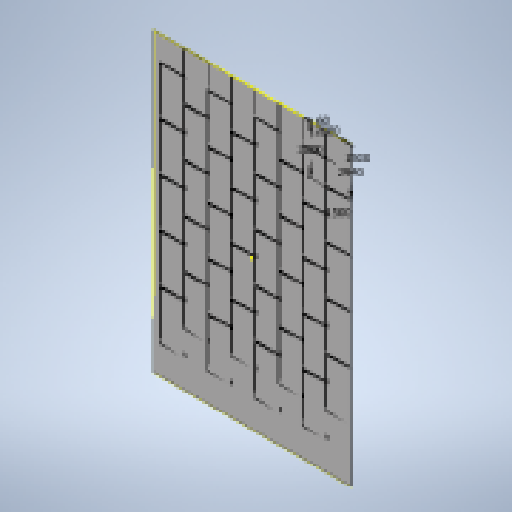
# Autodesk Inventor part: Part1
Saved by Autodesk Inventor 2026.2 (Build 302298000, 298)
## iProperties
Created: 2026-04-17
Part Number: Part1
Material: Generic
Document SubType Name: Sheet Metal
Designer: admin
Density: 1 g/cm^3
Sheet Metal Rule: Default_mm
Appearance: Default
Author: admin
Autodesk Inventor part; units mm, degrees
ref_plane "YZ Plane" through (0, 0, 0) normal (1, 0, 0) x (0, 1, 0)
ref_plane "XZ Plane" through (0, 0, 0) normal (0, 1, 0) x (-1, 0, 0)
ref_plane "XY Plane" through (0, 0, 0) normal (0, 0, 1) x (1, 0, 0)
sketch "Sketch1" plane through (0, 0, 0) normal (0, 0, 1) x (1, 0, 0)
  line L0 (6000, -9000) -> (-6000, -9000)
  line L1 (-6000, -9000) -> (-6000, 9000)
  line L2 (-6000, 9000) -> (6000, 9000)
  line L3 (6000, 9000) -> (6000, -9000)
  line L4 (6000, -9000) -> (-6000, 9000) construction
  line L5 (-6000, -9000) -> (6000, 9000) construction
  point P0 (0, 0)
  dimension "d0" = 12000
  dimension "d1" = 18000
  measures "d0" distance of L1.end L2.end
  measures "d1" distance of L0.end L1.end
extrude "Plate1" add sketch "Sketch1" along normal blind 6
sketch "Sketch2" plane through (0, 0, 6) normal (0, 0, 1) x (1, 0, 0)
  line L0 (6000, 9000) -> (6000, -9000)
  line L1 (-6000, 9000) -> (6000, 9000) projected
  line L2 (-6000, -9000) -> (-6000, 9000) projected
  line L3 (6000, -9000) -> (-6000, -9000) projected
  line L4 (5800, -8800) -> (5800, 8800)
  line L5 (5800, 8800) -> (-5800, 8800)
  line L6 (-5800, 8800) -> (-5800, -8800)
  line L7 (-5800, -8800) -> (5800, -8800)
  line L8 (6000, 9000) -> (-6000, 9000) projected
  line L9 (6000, 9000) -> (4500, 9000)
  line L10 (4500, 9000) -> (4500, 6000)
  line L11 (4500, 6000) -> (6000, 6000)
  line L12 (6000, 6000) -> (6000, 9000)
  line L13 (6000, -9000) -> (6000, 9000) projected
  line L14 (6000, 5975.1164) -> (4500, 5975.1164)
  line L15 (4500, 5975.1164) -> (4500, 2838.9347)
  line L16 (4500, 2838.9347) -> (6000, 2838.9347)
  line L17 (6000, 2838.9347) -> (6000, 5975.1164)
  line L18 (4448.9335, 7446.1559) -> (3367.2381, 7446.1559)
  line L19 (3367.2381, 7446.1559) -> (3367.2381, 4345.2957)
  line L20 (3367.2381, 4345.2957) -> (4448.9335, 4345.2957)
  line L21 (4448.9335, 4345.2957) -> (4448.9335, 7446.1559)
  line L22 (6000, 6064.0733) -> (4383.2518, 6064.0733) construction
  line L23 (4383.2518, 6064.0733) -> (4383.2518, 5895.7258) construction
  line L24 (4383.2518, 5895.7258) -> (6000, 5895.7258) construction
  line L25 (6000, 5895.7258) -> (6000, 6064.0733) construction
  line L26 (4383.2518, 5895.7258) -> (4569.2282, 5895.7258) construction
  line L27 (4569.2282, 5895.7258) -> (4569.2282, 4470.5931) construction
  line L28 (4569.2282, 4470.5931) -> (4383.2518, 4470.5931) construction
  line L29 (4383.2518, 4470.5931) -> (4383.2518, 5895.7258) construction
  line L30 (4448.9335, 9000) -> (3367.2381, 9000)
  line L31 (3367.2381, 9000) -> (3367.2381, 7500)
  line L32 (3367.2381, 7500) -> (4448.9335, 7500)
  line L33 (4448.9335, 7500) -> (4448.9335, 9000)
  line L34 (4569.2282, 7703.5758) -> (4383.2518, 7703.5758) construction
  line L35 (4383.2518, 7703.5758) -> (4383.2518, 6064.0733) construction
  line L36 (4383.2518, 6064.0733) -> (4569.2282, 6064.0733) construction
  line L37 (4569.2282, 6064.0733) -> (4569.2282, 7703.5758) construction
  dimension "d17" = 200
  dimension "d18" = 1500
  dimension "d19" = 3000
  constraints: 66 end point, 14 parallel, 7 horizontal, 7 perpendicular, 3 point on line, 3 other
  measures "d17" distance between parallel lines of L0 L4
  measures "d18" distance of L11.end L10.end
  measures "d19" distance of L10.end L9.end
equation "\"d2\" = Thickness"
equation "\"BendRadius\" = Thickness"
equation "\"BendReliefWidth\" = Thickness"
equation "\"BendReliefDepth\" = 0.5 * Thickness"
equation "\"CornerReliefSize\" = 4 * Thickness"
equation "\"MinimumRemnant\" = 2 * Thickness"
equation "\"TransitionRadius\" = BendRadius"
equation "\"JacobiRadiusSize\" = BendRadius"
equation "\"GapSize\" = Thickness"
equation "\"Thickness\" = 6"
body "Solid1"
